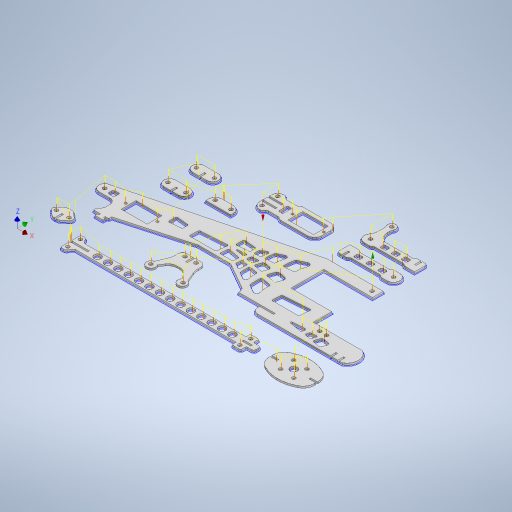
# Autodesk Inventor part: carbon_15
Saved by Autodesk Inventor 2024 (Build 280153000, 153)
## iProperties
Created: 2024-04-23
Part Number: carbon_15
Material: Generic
Document SubType Name: Modeling
Designer: nikop
Density: 1 g/cm^3
Appearance: Default
Author: nikop
Autodesk Inventor part; units mm, degrees
(part 1 of 2)
ref_plane "YZ Plane" through (0, 0, 0) normal (1, 0, 0) x (0, 1, 0)
ref_plane "XZ Plane" through (0, 0, 0) normal (0, 1, 0) x (-1, 0, 0)
ref_plane "XY Plane" through (0, 0, 0) normal (0, 0, 1) x (1, 0, 0)
sketch "Sketch2" plane through (0, 0, 0) normal (0, 1, 0) x (-1, 0, 0)
  line L0 (63.9659, -21.9846) -> (63.9659, -21.2726)
  line L1 (42.3159, -21.2726) -> (42.3159, -21.9846)
  arc A0 (42.3159, -21.9846) -> (48.3159, -27.9846) centre (48.3159, -21.9846) ccw
  line L2 (48.3159, -27.9846) -> (57.9659, -27.9846)
  arc A1 (57.9659, -27.9846) -> (63.9659, -21.9846) centre (57.9659, -21.9846) ccw
  line L3 (114.4342, 45.8312) -> (115.9235, 45.8312)
  line L4 (115.9235, 45.8312) -> (117.4264, 45.8275)
  line L5 (32.988, -58.0785) -> (33.7, -58.0785)
  arc A2 (33.7, -58.0785) -> (39.7, -52.0785) centre (33.7, -52.0785) ccw
  arc A3 (39.7, -42.4285) -> (33.7, -36.4285) centre (33.7, -42.4285) ccw
  line L6 (33.7, -36.4285) -> (32.988, -36.4285)
  line L7 (-8.55, -41.8285) -> (-8.55, -47.2535)
  line L8 (-8.55, -47.2535) -> (-8.55, -52.6785)
  line L9 (32.988, -58.0785) -> (31.0417, -56.1321)
  line L10 (-6.9772, -57.0785) -> (16.4833, -57.0785)
  line L11 (18.6047, -56.1998) -> (18.6723, -56.1321)
  line L12 (27.488, -55.2535) -> (28.9204, -55.2535)
  line L13 (27.488, -55.2535) -> (20.7936, -55.2535)
  line L14 (-12.85, -47.2535) -> (-12.85, -51.3363)
  line L15 (-11.5744, -54.265) -> (-9.7016, -56.0072)
  arc A4 (-12.85, -51.3363) -> (-11.5744, -54.265) centre (-8.85, -51.3363) ccw
  arc A5 (-9.7016, -56.0072) -> (-6.9772, -57.0785) centre (-6.9772, -53.0785) ccw
  arc A6 (31.0417, -56.1321) -> (28.9204, -55.2535) centre (28.9204, -58.2535) ccw
  arc A7 (20.7936, -55.2535) -> (18.6723, -56.1321) centre (20.7936, -58.2535) ccw
  arc A8 (16.4833, -57.0785) -> (18.6047, -56.1998) centre (16.4833, -54.0785) ccw
  line L16 (32.988, -36.4285) -> (31.0417, -38.3748)
  line L17 (-6.9772, -37.4285) -> (16.4833, -37.4285)
  line L18 (18.6047, -38.3071) -> (18.6723, -38.3748)
  line L19 (27.488, -39.2535) -> (28.9204, -39.2535)
  line L20 (27.488, -39.2535) -> (20.7936, -39.2535)
  line L21 (-12.85, -47.2535) -> (-12.85, -43.1706)
  line L22 (-11.5744, -40.2419) -> (-9.7016, -38.4997)
  arc A9 (-11.5744, -40.2419) -> (-12.85, -43.1706) centre (-8.85, -43.1706) ccw
  arc A10 (-6.9772, -37.4285) -> (-9.7016, -38.4997) centre (-6.9772, -41.4285) ccw
  arc A11 (28.9204, -39.2535) -> (31.0417, -38.3748) centre (28.9204, -36.2535) ccw
  arc A12 (18.6723, -38.3748) -> (20.7936, -39.2535) centre (20.7936, -36.2535) ccw
  arc A13 (18.6047, -38.3071) -> (16.4833, -37.4285) centre (16.4833, -40.4285) ccw
  line L23 (23.488, -51.2535) -> (21.55, -51.2535)
  line L24 (20.55, -50.2535) -> (20.55, -44.2535)
  line L25 (24.488, -50.2535) -> (24.488, -44.2535)
  line L26 (23.488, -43.2535) -> (21.55, -43.2535)
  arc A14 (23.488, -51.2535) -> (24.488, -50.2535) centre (23.488, -50.2535) ccw
  arc A15 (20.55, -50.2535) -> (21.55, -51.2535) centre (21.55, -50.2535) ccw
  arc A16 (21.55, -43.2535) -> (20.55, -44.2535) centre (21.55, -44.2535) ccw
  arc A17 (24.488, -44.2535) -> (23.488, -43.2535) centre (23.488, -44.2535) ccw
  arc A18 (-39.6917, -79.1119) -> (-39.0716, -76.4297) centre (-45.0715, -76.4553) ccw
  arc A19 (-39.6917, -79.1119) -> (-33.443, -79.1097) centre (-36.5668, -80.6883) ccw
  arc A20 (-34.0716, -76.4362) -> (-33.443, -79.1097) centre (-28.0716, -76.4362) ccw
  arc A21 (-32.1328, -65.5122) -> (-34.0716, -71.4122) centre (-24.1248, -71.4122) ccw
  arc A22 (-32.1328, -65.5122) -> (-36.5683, -56.76) centre (-36.5683, -62.26) ccw
  line L27 (-36.5683, -56.76) -> (-41.2399, -56.76)
  arc A23 (-41.2399, -56.76) -> (-42.6541, -57.3458) centre (-41.2399, -58.76) ccw
  line L28 (-42.6541, -57.3458) -> (-42.9825, -57.6743)
  arc A24 (-44.3967, -58.26) -> (-42.9825, -57.6743) centre (-44.3967, -56.26) ccw
  line L29 (-69.3967, -58.26) -> (-71.0483, -57.3065)
  arc A25 (-71.0483, -57.3065) -> (-72.5112, -56.805) centre (-72.378, -58.8005) ccw
  line L30 (-72.5112, -56.805) -> (-78.1828, -56.805)
  arc A26 (-72.5112, -67.805) -> (-71.097, -67.2192) centre (-72.5112, -65.805) ccw
  line L31 (-71.097, -67.2192) -> (-70.7686, -66.8907)
  arc A27 (-69.3967, -66.26) -> (-70.7686, -66.8907) centre (-69.309, -68.2581) ccw
  arc A28 (-42.9825, -66.8458) -> (-44.3967, -66.26) centre (-44.3967, -68.26) ccw
  line L32 (-42.9825, -66.8458) -> (-41.9972, -67.8311)
  arc A29 (-39.0716, -74.8989) -> (-41.9972, -67.8311) centre (-49.0716, -74.8989) ccw
  arc A30 (-68.7467, -39.07) -> (-67.3325, -39.6557) centre (-67.3325, -37.6557) ccw
  line L33 (-68.7467, -39.07) -> (-69.0752, -38.7415)
  arc A31 (-69.0752, -38.7415) -> (-70.4894, -38.1557) centre (-70.4894, -40.1557) ccw
  line L34 (-70.4894, -38.1557) -> (-75.1609, -38.1557)
  arc A32 (-75.1609, -38.1557) -> (-80.6609, -43.6557) centre (-75.1609, -43.6557) ccw
  arc A33 (-80.6609, -43.6557) -> (-75.1609, -49.1557) centre (-75.1609, -43.6557) ccw
  line L35 (-75.1609, -49.1557) -> (-70.4894, -49.1557)
  arc A34 (-70.4894, -49.1557) -> (-69.0752, -48.57) centre (-70.4894, -47.1557) ccw
  line L36 (-69.0752, -48.57) -> (-68.7467, -48.2415)
  arc A35 (-67.3325, -47.6557) -> (-68.7467, -48.2415) centre (-67.3325, -49.6557) ccw
  arc A36 (-41.2081, -48.1834) -> (-42.3325, -47.6557) centre (-42.578, -49.6406) ccw
  line L37 (-41.2081, -48.1834) -> (-40.8797, -48.5118)
  arc A37 (-40.8797, -48.5118) -> (-39.4655, -49.0976) centre (-39.4655, -47.0976) ccw
  line L38 (-39.4655, -49.0976) -> (-33.7939, -49.0976)
  arc A38 (-39.4655, -38.0976) -> (-40.8797, -38.6834) centre (-39.4655, -40.0976) ccw
  line L39 (-40.8797, -38.6834) -> (-41.2081, -39.0118)
  arc A39 (-42.3325, -39.6557) -> (-41.2081, -39.0118) centre (-42.7106, -37.6918) ccw
  line L40 (-56.1358, -62.2237) -> (-56.1358, -63.2237)
  line L41 (-56.1358, -62.2237) -> (-56.1358, -61.2237)
  line L42 (-69.7689, -62.305) -> (-69.7689, -63.305)
  line L43 (-69.7689, -62.305) -> (-69.7689, -61.305)
  line L44 (-65.7689, -60.305) -> (-68.7689, -60.305)
  line L45 (-80.1828, -62.305) -> (-80.1828, -65.805)
  line L46 (-80.1828, -62.305) -> (-80.1828, -58.805)
  arc A40 (-80.1828, -65.805) -> (-78.1828, -67.805) centre (-78.1828, -65.805) ccw
  arc A41 (-69.7689, -63.305) -> (-68.7689, -64.305) centre (-68.7689, -63.305) ccw
  arc A42 (-68.7689, -60.305) -> (-69.7689, -61.305) centre (-68.7689, -61.305) ccw
  arc A43 (-57.1358, -64.2237) -> (-56.1358, -63.2237) centre (-57.1358, -63.2237) ccw
  arc A44 (-56.1358, -61.2237) -> (-57.1358, -60.2237) centre (-57.1358, -61.2237) ccw
  line L47 (-68.7689, -64.305) -> (-65.7689, -64.305)
  line L48 (-64.7689, -61.305) -> (-64.7689, -63.305)
  line L49 (-61.1358, -61.2237) -> (-61.1358, -63.2237)
  line L50 (-60.1358, -64.2237) -> (-57.1358, -64.2237)
  line L51 (-60.1358, -60.2237) -> (-57.1358, -60.2237)
  arc A45 (-65.7689, -64.305) -> (-64.7689, -63.305) centre (-65.7689, -63.305) ccw
  arc A46 (-64.7689, -61.305) -> (-65.7689, -60.305) centre (-65.7689, -61.305) ccw
  arc A47 (-61.1358, -63.2237) -> (-60.1358, -64.2237) centre (-60.1358, -63.2237) ccw
  arc A48 (-60.1358, -60.2237) -> (-61.1358, -61.2237) centre (-60.1358, -61.2237) ccw
  line L52 (-31.7939, -43.5976) -> (-31.7939, -40.0976)
  line L53 (-31.7939, -43.5976) -> (-31.7939, -47.0976)
  arc A49 (-31.7939, -40.0976) -> (-33.7939, -38.0976) centre (-33.7939, -40.0976) ccw
  line L54 (-67.9654, -43.7185) -> (-67.9654, -42.7185)
  line L55 (-67.9654, -43.7185) -> (-67.9654, -44.7185)
  line L56 (-42.268, -43.5976) -> (-42.268, -42.5976)
  line L57 (-42.268, -43.5976) -> (-42.268, -44.5976)
  line L58 (-46.268, -45.5976) -> (-43.268, -45.5976)
  arc A50 (-42.268, -42.5976) -> (-43.268, -41.5976) centre (-43.268, -42.5976) ccw
  arc A51 (-43.268, -45.5976) -> (-42.268, -44.5976) centre (-43.268, -44.5976) ccw
  arc A52 (-66.9654, -41.7185) -> (-67.9654, -42.7185) centre (-66.9654, -42.7185) ccw
  arc A53 (-67.9654, -44.7185) -> (-66.9654, -45.7185) centre (-66.9654, -44.7185) ccw
  line L59 (-43.268, -41.5976) -> (-46.268, -41.5976)
  line L60 (-47.268, -44.5976) -> (-47.268, -42.5976)
  line L61 (-62.9654, -44.7185) -> (-62.9654, -42.7185)
  line L62 (-63.9654, -41.7185) -> (-66.9654, -41.7185)
  line L63 (-63.9654, -45.7185) -> (-66.9654, -45.7185)
  arc A54 (-46.268, -41.5976) -> (-47.268, -42.5976) centre (-46.268, -42.5976) ccw
  arc A55 (-47.268, -44.5976) -> (-46.268, -45.5976) centre (-46.268, -44.5976) ccw
  arc A56 (-62.9654, -42.7185) -> (-63.9654, -41.7185) centre (-63.9654, -42.7185) ccw
  arc A57 (-63.9654, -45.7185) -> (-62.9654, -44.7185) centre (-63.9654, -44.7185) ccw
  line L64 (-63.4368, 73.5321) -> (-63.4368, 73.3321)
  arc A58 (-64.4368, 72.3321) -> (-63.4368, 73.3321) centre (-64.4368, 73.3321) ccw
  line L65 (-64.4368, 72.3321) -> (-67.9559, 72.3321)
  arc A59 (-67.9559, 72.3321) -> (-69.9559, 70.3321) centre (-67.9559, 70.3321) ccw
  line L66 (-69.9559, 70.3321) -> (-69.9559, 68.3321)
  arc A60 (-69.9559, 68.3321) -> (-67.9559, 66.3321) centre (-67.9559, 68.3321) ccw
  line L67 (-67.9559, 66.3321) -> (-64.4368, 66.3321)
  arc A61 (-63.4193, 65.3322) -> (-64.4368, 66.3321) centre (-64.4193, 65.3322) ccw
  line L68 (-63.4193, 65.3322) -> (-63.4193, 65.1321)
  line L69 (121.1391, 17.6529) -> (121.1391, 17.654)
  line L70 (4.289, 17.6186) -> (-16.8908, 29.6804)
  line L71 (105.5881, 35.3778) -> (105.5881, 34.2063)
  arc A62 (116.9799, 9.8778) -> (121.9799, 14.8778) centre (116.9799, 14.8778) ccw
  line L72 (105.0881, 35.8778) -> (99.4807, 35.8778)
  line L73 (95.4807, 37.4038) -> (94.2807, 37.4038)
  line L74 (100.6807, 37.4038) -> (99.4807, 37.4038)
  line L75 (93.9807, 37.7038) -> (93.9807, 39.1038)
  line L76 (100.9807, 37.7038) -> (100.9807, 39.1038)
  line L77 (95.4791, 37.4038) -> (94.2791, 37.4028)
  arc A63 (93.9807, 37.7038) -> (94.2807, 37.4038) centre (94.2807, 37.7038) ccw
  arc A64 (94.2807, 39.4038) -> (93.9807, 39.1038) centre (94.2807, 39.1038) ccw
  arc A65 (100.9807, 39.1038) -> (100.6807, 39.4038) centre (100.6807, 39.1038) ccw
  arc A66 (100.6807, 37.4038) -> (100.9807, 37.7038) centre (100.6807, 37.7038) ccw
  arc A67 (121.9799, 14.8778) -> (116.9799, 19.8778) centre (116.9799, 14.8778) ccw
  line L78 (116.9799, 19.8778) -> (107.4799, 19.8778)
  line L79 (105.5881, 35.3778) -> (105.5881, 34.8778)
  line L80 (105.0023, 32.792) -> (103.9444, 31.7341)
  line L81 (102.4799, 24.8778) -> (102.4799, 28.1985)
  arc A68 (103.9444, 31.7341) -> (102.4799, 28.1985) centre (107.4799, 28.1985) ccw
  arc A69 (102.4799, 24.8778) -> (107.4799, 19.8778) centre (107.4799, 24.8778) ccw
  arc A70 (105.0023, 32.792) -> (105.5881, 34.2063) centre (103.5881, 34.2063) ccw
  line L82 (92.4791, 35.3778) -> (92.4791, 33.2966)
  line L83 (92.9791, 35.8778) -> (95.4791, 35.8778)
  arc A71 (92.9791, 35.8778) -> (92.4791, 35.3778) centre (92.9791, 35.3778) ccw
  arc A72 (105.5881, 35.3778) -> (105.0881, 35.8778) centre (105.0881, 35.3778) ccw
  arc A73 (-19.2582, 33.8243) -> (-16.8908, 29.6804) centre (-14.2593, 33.9319) ccw
  arc A74 (112.0363, 15.6265) -> (112.0363, 14.1292) centre (116.9799, 14.8778) ccw
  line L84 (-9.9813, 1.6568) -> (-13.6957, 2.4536)
  arc A75 (-15.0721, 5.2892) -> (-13.7944, 8.5218) centre (-34.7824, 14.9487) ccw
  arc A76 (4.289, 17.6186) -> (6.789, 16.9487) centre (6.789, 21.9487) ccw
  arc A77 (-15.0721, 5.2892) -> (-13.6957, 2.4536) centre (-13.2762, 4.4091) ccw
  arc A78 (-10.6169, 22.7604) -> (-13.5514, 20.5207) centre (-11.6169, 21.0284) ccw
  line L85 (110.663, 17.3471) -> (107.4546, 17.5827)
  arc A79 (110.663, 12.4086) -> (112.0363, 14.1292) centre (110.5532, 13.9046) ccw
  arc A80 (112.0363, 15.6265) -> (110.663, 17.3471) centre (110.5532, 15.8511) ccw
  line L86 (110.663, 12.4086) -> (107.4546, 12.173)
  arc A81 (107.4546, 17.5827) -> (106.3814, 16.5854) centre (107.3814, 16.5854) ccw
  arc A82 (106.3814, 13.1703) -> (107.4546, 12.173) centre (107.3814, 13.1703) ccw
  line L87 (110.663, 12.4086) -> (107.4546, 12.173)
  line L88 (-8.4093, 1.7319) -> (-9.6983, 1.6372)
  line L89 (-8.4093, 1.7319) -> (-9.6983, 1.6372)
  line L90 (0.9741, 2.4209) -> (-3.375, 2.1015)
  line L91 (0.9741, 2.4209) -> (-3.375, 2.1015)
  line L92 (0.9741, 2.4209) -> (-3.375, 2.1015)
  line L93 (0.9741, 2.4209) -> (-3.375, 2.1015)
  line L94 (0.9741, 2.4209) -> (-3.375, 2.1015)
  line L95 (0.9741, 2.4209) -> (-3.375, 2.1015)
  line L96 (0.9741, 2.4209) -> (-3.375, 2.1015)
  line L97 (0.9741, 2.4209) -> (-3.375, 2.1015)
  line L98 (0.9741, 2.4209) -> (-3.375, 2.1015)
  line L99 (0.9741, 2.4209) -> (-3.375, 2.1015)
  line L100 (-8.4093, 1.7319) -> (-9.6983, 1.6372)
  line L101 (-8.4093, 1.7319) -> (-9.6983, 1.6372)
  line L102 (-8.4093, 1.7319) -> (-9.6983, 1.6372)
  line L103 (-8.4093, 1.7319) -> (-9.6983, 1.6372)
  line L104 (-8.4093, 1.7319) -> (-9.6983, 1.6372)
  line L105 (-8.4093, 1.7319) -> (-9.6983, 1.6372)
  line L106 (-8.4093, 1.7319) -> (-9.6983, 1.6372)
  line L107 (-8.4093, 1.7319) -> (-9.6983, 1.6372)
  line L108 (16.896, 3.5901) -> (16.8305, 3.5853)
  line L109 (16.896, 3.5901) -> (16.8305, 3.5853)
  line L110 (16.896, 3.5901) -> (16.8305, 3.5853)
  line L111 (16.896, 3.5901) -> (16.8305, 3.5853)
  line L112 (16.896, 3.5901) -> (16.8305, 3.5853)
  line L113 (16.896, 3.5901) -> (16.8305, 3.5853)
  line L114 (16.896, 3.5901) -> (16.8305, 3.5853)
  line L115 (16.896, 3.5901) -> (16.8305, 3.5853)
  line L116 (16.896, 3.5901) -> (16.8305, 3.5853)
  line L117 (13.1011, 3.3114) -> (6.3051, 2.8124)
  line L118 (43.3602, 5.5334) -> (25.7785, 4.2424)
  line L119 (43.3602, 5.5334) -> (25.7785, 4.2424)
  line L120 (43.3602, 5.5334) -> (25.7785, 4.2424)
  line L121 (43.3602, 5.5334) -> (25.7785, 4.2424)
  line L122 (43.3602, 5.5334) -> (25.7785, 4.2424)
  line L123 (43.3602, 5.5334) -> (25.7785, 4.2424)
  line L124 (43.3602, 5.5334) -> (25.7785, 4.2424)
  line L125 (43.3602, 5.5334) -> (25.7785, 4.2424)
  line L126 (43.3602, 5.5334) -> (25.7785, 4.2424)
  line L127 (43.3602, 5.5334) -> (21.4119, 3.9217)
  line L128 (6.6161, 5.5458) -> (13.1579, 4.3013)
  line L129 (-2.2448, 7.2316) -> (1.6945, 6.4821)
  line L130 (-12.6513, 9.2114) -> (-6.6798, 8.0753)
  line L131 (7.1768, 8.493) -> (16.5175, 6.7159)
  line L132 (-1.6841, 10.1787) -> (2.2552, 9.4293)
  line L133 (-12.0906, 12.1585) -> (-6.1191, 11.0225)
  arc A83 (-12.9006, 13.2197) -> (-13.5514, 20.5207) centre (-34.7824, 14.9487) ccw
  arc A84 (-12.9006, 13.2197) -> (-12.0906, 12.1585) centre (-11.9037, 13.1409) ccw
  arc A85 (-12.6513, 9.2114) -> (-13.7944, 8.5218) centre (-12.8382, 8.229) ccw
  arc A86 (-5.9041, 6.8221) -> (-6.6798, 8.0753) centre (-6.8667, 7.093) ccw
  arc A87 (-9.9813, 1.6568) -> (-9.6983, 1.6372) centre (-9.7716, 2.6345) ccw
  arc A88 (-8.4093, 1.7319) -> (-7.5757, 2.3078) centre (-8.4826, 2.7292) ccw
  arc A89 (-4.3836, 3.4526) -> (-3.375, 2.1015) centre (-3.4482, 3.0989) ccw
  arc A90 (-2.2448, 7.2316) -> (-3.3974, 6.5089) centre (-2.4317, 6.2492) ccw
  arc A91 (2.4754, 5.2478) -> (1.6945, 6.4821) centre (1.5076, 5.4998) ccw
  arc A92 (0.9741, 2.4209) -> (1.8524, 3.1107) centre (0.9009, 3.4182) ccw
  arc A93 (5.2668, 4.0718) -> (6.3051, 2.8124) centre (6.2319, 3.8097) ccw
  arc A94 (6.6161, 5.5458) -> (5.4595, 4.8078) centre (6.4292, 4.5635) ccw
  arc A95 (-2.4908, 11.2742) -> (-1.6841, 10.1787) centre (-1.4972, 11.1611) ccw
  arc A96 (2.2552, 9.4293) -> (3.4347, 10.2907) centre (2.4421, 10.4117) ccw
  arc A97 (3.7029, 13.8877) -> (3.2033, 14.7813) centre (2.7033, 13.9153) ccw
  arc A98 (-0.807, 17.0967) -> (-2.3062, 16.1924) centre (-1.307, 16.2306) ccw
  arc A99 (-5.0732, 19.1157) -> (-5.5636, 19.8429) centre (-6.0636, 18.9768) ccw
  arc A100 (7.6705, 13.9487) -> (6.6716, 12.9958) centre (7.6705, 12.9487) ccw
  arc A101 (18.166, 12.9067) -> (17.1668, 13.9487) centre (17.1668, 12.9487) ccw
  arc A102 (16.5175, 6.7159) -> (17.6954, 7.565) centre (16.7044, 7.6983) ccw
  arc A103 (-6.1191, 11.0225) -> (-4.9374, 11.9034) centre (-5.9322, 12.0049) ccw
  arc A104 (13.1011, 3.3114) -> (13.1579, 4.3013) centre (13.0644, 3.8101) ccw
  line L134 (13.1011, 3.3114) -> (6.3051, 2.8124)
  line L135 (13.1011, 3.3114) -> (6.3051, 2.8124)
  line L136 (13.1011, 3.3114) -> (6.3051, 2.8124)
  line L137 (13.1011, 3.3114) -> (6.3051, 2.8124)
  line L138 (13.1011, 3.3114) -> (6.3051, 2.8124)
  line L139 (13.1011, 3.3114) -> (6.3051, 2.8124)
  line L140 (13.1011, 3.3114) -> (6.3051, 2.8124)
  line L141 (13.1011, 3.3114) -> (6.3051, 2.8124)
  line L142 (13.1011, 3.3114) -> (6.3051, 2.8124)
  line L143 (23.709, 13.9487) -> (22.1709, 13.9487)
  line L144 (17.1668, 13.9487) -> (7.6705, 13.9487)
  arc A105 (6.372, 9.6041) -> (7.1768, 8.493) centre (7.3637, 9.4754) ccw
  line L145 (43.6933, 13.9487) -> (23.709, 13.9487)
  arc A106 (22.1709, 13.9487) -> (21.1717, 12.9873) centre (22.1709, 12.9487) ccw
  arc A107 (20.3528, 5.0861) -> (21.4119, 3.9217) centre (21.3387, 4.919) ccw
  arc A108 (43.3602, 5.5334) -> (44.2818, 6.4287) centre (43.287, 6.5307) ccw
  arc A109 (44.693, 12.9245) -> (43.6933, 13.9487) centre (43.6933, 12.9487) ccw
  line L146 (3.2033, 14.7813) -> (-0.807, 17.0967)
  line L147 (-5.5636, 19.8429) -> (-10.6169, 22.7604)
  line L148 (106.3814, 16.5854) -> (106.3814, 13.1703)
  arc A110 (-7.5757, 2.3078) -> (-5.9041, 6.8221) centre (-34.7824, 14.9487) ccw
  arc A111 (-4.9374, 11.9034) -> (-5.0732, 19.1157) centre (-34.7824, 14.9487) ccw
  arc A112 (-4.3836, 3.4526) -> (-3.3974, 6.5089) centre (-34.7824, 14.9487) ccw
  arc A113 (-2.4908, 11.2742) -> (-2.3062, 16.1924) centre (-34.7824, 14.9487) ccw
  arc A114 (17.6954, 7.565) -> (18.166, 12.9067) centre (-40.2824, 15.3634) ccw
  arc A115 (20.3528, 5.0861) -> (21.1717, 12.9873) centre (-40.2824, 15.3634) ccw
  arc A116 (21.185, 17.3634) -> (21.1834, 17.4134) centre (-40.2824, 15.3634) ccw
  arc A117 (44.2818, 6.4287) -> (44.693, 12.9245) centre (-38.7824, 14.9487) ccw
  arc A118 (47.6944, 16.9717) -> (47.6935, 17.007) centre (-38.7825, 14.9717) ccw
  arc A119 (1.8524, 3.1107) -> (2.4754, 5.2478) centre (-34.7824, 14.9487) ccw
  arc A120 (3.4347, 10.2907) -> (3.7029, 13.8877) centre (-34.7824, 14.9487) ccw
  arc A121 (3.7148, 14.486) -> (3.7149, 14.4939) centre (-34.7824, 14.9487) ccw
  arc A122 (5.2668, 4.0718) -> (5.4595, 4.8078) centre (-34.7824, 14.9487) ccw
  arc A123 (6.372, 9.6041) -> (6.6716, 12.9958) centre (-34.7824, 14.9487) ccw
  line L149 (18.1699, 45.3626) -> (15.4569, 49.3848)
  line L150 (33.8183, 45.3626) -> (36.5313, 49.3848)
  line L151 (25.9941, 41.8361) -> (24.8022, 41.8361)
  line L152 (25.9941, 41.8361) -> (27.186, 41.8361)
  arc A124 (18.1699, 45.3626) -> (24.8022, 41.8361) centre (24.8022, 49.8361) ccw
  arc A125 (27.186, 41.8361) -> (33.8183, 45.3626) centre (27.186, 49.8361) ccw
  circle A126 centre (11.9941, 51.8361) radius 1.55
  circle A127 centre (39.9941, 51.8361) radius 1.55
  line L153 (94.2807, 39.4038) -> (100.6807, 39.4038)
  line L154 (-19.2582, 33.9482) -> (-19.2582, 33.8243)
  line L155 (89.0441, 65.8321) -> (89.3041, 65.8321) construction
  line L156 (92.0263, 66.8987) -> (92.0263, 61.3987)
  arc A128 (89.5263, 60.3987) -> (92.0263, 61.3987) centre (89.7806, 63.3879) ccw
  arc A129 (87.0263, 61.3987) -> (89.5263, 60.3987) centre (89.272, 63.3879) ccw
  line L157 (92.0419, 71.8659) -> (92.0419, 77.3659)
  arc A130 (92.0419, 77.3659) -> (89.5419, 78.3659) centre (89.7962, 75.3767) ccw
  arc A131 (89.5419, 78.3659) -> (87.0263, 77.3481) centre (89.2876, 75.3767) ccw
  arc A132 (119.3083, 58.1434) -> (117.4289, 58.8275) centre (117.4012, 55.8276) ccw
  arc A133 (117.4264, 45.8275) -> (119.3058, 46.5115) centre (117.3988, 48.8273) ccw
  arc A134 (114.4127, 58.8312) -> (112.5333, 58.1472) centre (114.4404, 55.8313) ccw
  arc A135 (112.5549, 46.5152) -> (114.4342, 45.8312) centre (114.4619, 48.8311) ccw
  line L158 (-55.8664, 73.4812) -> (84.1336, 73.4812)
  line L159 (-55.8758, 65.1984) -> (84.1242, 65.1984)
  line L160 (83.9404, -12.0118) -> (84.7029, -12.0118)
  line L161 (87.7029, -12.0118) -> (88.4653, -12.0118)
  circle A136 centre (89.0441, 74.8321) radius 1.55
  circle A137 centre (89.0441, 63.8321) radius 1.55
  arc A138 (87.0263, 61.3987) -> (84.1242, 65.1984) centre (79.508, 58.6647) ccw
  arc A139 (84.1336, 73.4812) -> (87.0263, 77.3481) centre (79.4727, 79.9832) ccw
  circle A140 centre (-59.4485, 74.0821) radius 1.55
  circle A141 centre (-59.4562, 64.5821) radius 1.55
  line L162 (-63.4193, 65.1321) -> (-63.4193, 62.1321)
  arc A142 (-63.4193, 62.1321) -> (-61.5716, 61.3667) centre (-61.8326, 63.3496) ccw
  line L163 (-55.8758, 65.1984) -> (-55.8758, 62.1321)
  arc A143 (-57.7235, 61.3667) -> (-55.8758, 62.1321) centre (-57.4625, 63.3496) ccw
  line L164 (-61.5716, 61.3667) -> (-57.7235, 61.3667)
  line L165 (-63.4368, 73.5321) -> (-63.4368, 76.5321)
  line L166 (-55.8664, 73.4812) -> (-55.8664, 76.5321)
  arc A144 (-55.8664, 76.5321) -> (-57.7142, 77.2974) centre (-57.4531, 75.3146) ccw
  arc A145 (-61.589, 77.2974) -> (-63.4368, 76.5321) centre (-61.8501, 75.3146) ccw
  line L167 (-61.589, 77.2974) -> (-57.7142, 77.2974)
  circle A146 centre (21.2441, 31.3361) radius 1.55
  circle A147 centre (30.7441, 31.3361) radius 1.55
  line L168 (24.4941, 28.3361) -> (19.4941, 28.3361)
  arc A148 (15.9585, 31.8717) -> (19.4941, 28.3361) centre (19.9343, 32.3118) ccw
  line L169 (15.9585, 31.8717) -> (15.9585, 34.8717)
  arc A149 (15.9585, 34.8717) -> (14.9831, 39.7756) centre (5.9744, 35.4347) ccw
  line L170 (14.9831, 39.7756) -> (11.5389, 48.0905)
  arc A150 (15.4569, 49.3848) -> (11.5389, 48.0905) centre (12.423, 51.9916) ccw
  circle A151 centre (110.4234, 52.3502) radius 1.55
  circle A152 centre (121.4236, 52.3589) radius 1.55
  line L171 (112.5333, 58.1472) -> (107.937, 54.2904)
  line L172 (112.5549, 46.5152) -> (107.9586, 50.372)
  arc A153 (107.937, 54.2904) -> (107.9586, 50.372) centre (109.5006, 52.3397) ccw
  line L173 (119.3058, 46.5115) -> (123.9021, 50.3682)
  line L174 (119.3083, 58.1434) -> (123.9045, 54.2867)
  arc A154 (123.9021, 50.3682) -> (123.9045, 54.2867) centre (122.3504, 52.3284) ccw
  line L175 (39.7, -52.0785) -> (39.7, -51.7535)
  line L176 (-8.55, -52.6785) -> (-8.55, -53.6785)
  line L177 (-8.55, -41.8285) -> (-8.55, -40.8285)
  line L178 (-8.55, -53.6785) -> (13.65, -53.6785)
  line L179 (-8.55, -40.8285) -> (13.65, -40.8285)
  line L180 (13.65, -53.6785) -> (13.65, -40.8285)
  line L181 (39.7, -42.4285) -> (39.7, -42.7535)
  line L182 (39.7, -48.7535) -> (39.7, -45.7535)
  circle A155 centre (35.788, -40.3535) radius 1.55
  circle A156 centre (35.788, -54.1535) radius 1.55
  circle A157 centre (46.2409, -24.0726) radius 1.55
  circle A158 centre (60.0409, -24.0726) radius 1.55
  line L183 (-72.5112, -67.805) -> (-73.6828, -67.805)
  line L184 (-76.6797, -67.805) -> (-78.1828, -67.805)
  circle A159 centre (-36.5683, -62.26) radius 1.55
  circle A160 centre (-36.5748, -80.6723) radius 1.55
  circle A161 centre (-75.1609, -43.6557) radius 1.55
  line L185 (-33.7939, -38.0976) -> (-35.2939, -38.0976)
  line L186 (-38.2939, -38.0976) -> (-39.4655, -38.0976)
  line L187 (94.0577, 10.5517) -> (71.558, 10.6609)
  line L188 (94.0577, 10.5517) -> (94.0577, 23.4561)
  line L189 (94.0577, 23.4561) -> (71.5577, 23.4556)
  line L190 (71.5577, 23.4556) -> (71.558, 10.6609)
  circle A162 centre (116.9704, 14.938) radius 1.55
  line L191 (-34.0716, -76.4362) -> (-34.0716, -71.4122)
  line L192 (-39.0716, -76.4297) -> (-39.0716, -74.8989)
  circle A163 centre (-106.6787, 63.0954) radius 1.525
  circle A164 centre (-95.365, 74.4091) radius 1.525
  circle A165 centre (-107.7394, 75.4697) radius 1.525
  circle A166 centre (-94.3044, 62.0347) radius 1.525
  line L193 (-44.3967, -66.26) -> (-69.3967, -66.26)
  line L194 (-44.3967, -58.26) -> (-69.3967, -58.26)
  line L195 (-51.7166, -61.152) -> (-51.7166, -63.152)
  line L196 (-50.7166, -60.152) -> (-47.7166, -60.152)
  line L197 (-50.7166, -64.152) -> (-47.7166, -64.152)
  arc A167 (-51.7166, -63.152) -> (-50.7166, -64.152) centre (-50.7166, -63.152) ccw
  arc A168 (-50.7166, -60.152) -> (-51.7166, -61.152) centre (-50.7166, -61.152) ccw
  arc A169 (-47.7166, -64.152) -> (-46.7166, -63.152) centre (-47.7166, -63.152) ccw
  line L198 (-46.7166, -62.152) -> (-46.7166, -63.152)
  line L199 (-46.7166, -62.152) -> (-46.7166, -61.152)
  arc A170 (-46.7166, -61.152) -> (-47.7166, -60.152) centre (-47.7166, -61.152) ccw
  line L200 (-67.3325, -47.6557) -> (-42.3325, -47.6557)
  line L201 (-67.3325, -39.6557) -> (-42.3325, -39.6557)
  line L202 (-52.5769, -43.6799) -> (-52.5769, -42.6799)
  line L203 (-53.5769, -41.6799) -> (-56.5769, -41.6799)
  line L204 (-52.5769, -43.6799) -> (-52.5769, -44.6799)
  arc A171 (-53.5769, -45.6799) -> (-52.5769, -44.6799) centre (-53.5769, -44.6799) ccw
  arc A172 (-52.5769, -42.6799) -> (-53.5769, -41.6799) centre (-53.5769, -42.6799) ccw
  line L205 (-57.5769, -44.6799) -> (-57.5769, -42.6799)
  arc A173 (-57.5769, -44.6799) -> (-56.5769, -45.6799) centre (-56.5769, -44.6799) ccw
  arc A174 (-56.5769, -41.6799) -> (-57.5769, -42.6799) centre (-56.5769, -42.6799) ccw
  line L206 (-56.5769, -45.6799) -> (-53.5769, -45.6799)
  line L207 (-75.2523, 42.9487) -> (-99.2523, 42.9487)
  line L208 (-74.2523, 25.0966) -> (-115.3023, 25.0966)
  line L209 (83.9404, -12.0118) -> (79.9404, -12.0118)
  line L210 (88.4653, -12.0118) -> (92.4653, -12.0118)
  line L211 (88.4653, -12.0118) -> (92.4653, -12.0118) construction
  circle A175 centre (78.4154, -17.0118) radius 1.525
  arc A176 (79.9404, -12.0118) -> (79.9404, -22.0118) centre (79.9404, -17.0118) ccw
  line L212 (79.9404, -22.0118) -> (92.4653, -22.0118)
  arc A177 (92.4653, -22.0118) -> (92.4653, -12.0118) centre (92.4653, -17.0118) ccw
  circle A178 centre (93.9903, -17.0118) radius 1.525
  line L213 (42.3159, -21.2726) -> (42.3159, -19.7726)
  line L214 (63.9659, -21.2726) -> (63.9659, -19.7726)
  line L215 (42.3159, -19.7726) -> (63.9659, -19.7726)
  line L216 (6.789, 16.9487) -> (33.789, 16.9487)
  line L217 (-50.9967, 34.8873) -> (-19.2582, 34.8873)
  line L218 (-19.2582, 34.8873) -> (-19.2582, 33.8243)
  arc A179 (-87.2534, 57.9059) -> (-81.2534, 67.2522) centre (-91.2517, 67.0718) ccw
  arc A180 (-120.7904, 67.2522) -> (-114.7904, 57.9059) centre (-110.792, 67.0718) ccw
  arc A181 (-114.7904, 57.9059) -> (-87.2534, 57.9059) centre (-101.0219, 84.5598) ccw
  arc A182 (-81.2534, 70.2522) -> (-87.2534, 79.5985) centre (-91.2517, 70.4327) ccw
  arc A183 (-114.7904, 79.5985) -> (-120.7904, 70.2522) centre (-110.792, 70.4327) ccw
  arc A184 (-87.2534, 79.5985) -> (-114.7904, 79.5985) centre (-101.0219, 52.9447) ccw
  line L219 (-26.9701, 15.6496) -> (-19.8043, 14.2863)
  arc A185 (-18.5493, 23.9983) -> (-19.1376, 24.8708) centre (-19.7376, 23.8316) ccw
  arc A186 (-19.8043, 14.2863) -> (-18.3863, 15.3434) centre (-19.5801, 15.4652) ccw
  arc A187 (-18.3863, 15.3434) -> (-18.5493, 23.9983) centre (-54.2003, 18.9978) ccw
  line L220 (-19.1376, 24.8708) -> (-25.2017, 28.3719)
  arc A188 (-27.9421, 16.923) -> (-26.9701, 15.6496) centre (-26.7459, 16.8285) ccw
  arc A189 (-27.9421, 16.923) -> (-28.7231, 25.6842) centre (-54.2003, 18.9978) ccw
  arc A190 (-25.2017, 28.3719) -> (-28.7231, 25.6842) centre (-26.4017, 26.2934) ccw
  line L221 (-21.5647, 2.7268) -> (-23.1115, 2.6132)
  line L222 (-21.5647, 2.7268) -> (-23.1115, 2.6132)
  line L223 (-21.5647, 2.7268) -> (-23.1115, 2.6132)
  line L224 (-21.5647, 2.7268) -> (-23.1115, 2.6132)
  line L225 (-26.6551, 11.7022) -> (-19.4892, 10.339)
  line L226 (-21.5647, 2.7268) -> (-23.1115, 2.6132)
  line L227 (-23.451, 2.6367) -> (-27.9083, 3.5928)
  arc A191 (-29.56, 6.9956) -> (-27.9083, 3.5928) centre (-27.4049, 5.9395) ccw
  arc A192 (-29.56, 6.9956) -> (-28.0267, 10.8747) centre (-53.2124, 18.587) ccw
  line L228 (-21.5647, 2.7268) -> (-23.1115, 2.6132)
  line L229 (-21.5647, 2.7268) -> (-23.1115, 2.6132)
  line L230 (-21.5647, 2.7268) -> (-23.1115, 2.6132)
  line L231 (-21.5647, 2.7268) -> (-23.1115, 2.6132)
  line L232 (-21.5647, 2.7268) -> (-23.1115, 2.6132)
  arc A193 (-20.5643, 3.4179) -> (-18.5584, 8.835) centre (-53.2124, 18.587) ccw
  arc A194 (-21.5647, 2.7268) -> (-20.5643, 3.4179) centre (-21.6525, 3.9236) ccw
  arc A195 (-18.5584, 8.835) -> (-19.4892, 10.339) centre (-19.7135, 9.1601) ccw
  arc A196 (-23.451, 2.6367) -> (-23.1115, 2.6132) centre (-23.1993, 3.81) ccw
  arc A197 (-26.6551, 11.7022) -> (-28.0267, 10.8747) centre (-26.8793, 10.5234) ccw
  circle A198 centre (-101.0219, 68.7522) radius 3
  line L233 (-74.2523, 25.0966) -> (-81.7523, 25.0966)
  line L234 (-74.2523, 25.0966) -> (-81.7523, 25.0966)
  line L235 (-78.1828, -56.805) -> (-80.1828, -56.805)
  line L236 (-80.1828, -56.805) -> (-80.1828, -58.805)
  line L237 (-33.7939, -49.0976) -> (-31.7939, -49.0976)
  line L238 (-33.7939, -49.0976) -> (-35.7939, -49.0976) construction
  line L239 (-31.7939, -49.0976) -> (-31.7939, -47.0976)
  arc A199 (-38.9967, 37.8873) -> (-44.058, 42.9487) centre (-43.9963, 37.9491) ccw
  line L240 (-75.2523, 42.9487) -> (-44.058, 42.9487)
  line L241 (-73.7828, -67.805) -> (-73.6828, -67.805)
  line L242 (-76.5828, -67.805) -> (-76.6797, -67.805)
  line L243 (-38.1939, -38.0976) -> (-38.2939, -38.0976)
  line L244 (-35.3939, -38.0976) -> (-35.2939, -38.0976)
  line L245 (-101.2523, 42.9487) -> (-99.2523, 42.9487)
  circle A200 centre (-89.7523, 29.0966) radius 1.525
  circle A201 centre (-83.7523, 29.0966) radius 1.525
  line L246 (-101.2523, 42.9487) -> (-99.2523, 42.9487) construction
  circle A202 centre (16.1, -47.2535) radius 1.05
  circle A203 centre (-11, -47.2535) radius 1.05
  line L247 (-101.2523, 42.9487) -> (-105.2523, 42.9487)
  line L248 (-101.2523, 42.9487) -> (-97.2523, 42.9487) construction
  line L249 (-108.2523, 37.9487) -> (-108.2523, 42.9487)
  line L250 (-108.2523, 42.9487) -> (-113.2523, 42.9487)
  line L251 (-113.2523, 42.9487) -> (-113.2523, 37.9487)
  line L252 (-115.2523, 42.9487) -> (-117.2523, 42.9487)
  line L253 (-115.3023, 25.0966) -> (-116.7523, 25.0966)
  arc A204 (-117.2523, 42.9487) -> (-116.7523, 25.0966) centre (-112.5027, 34.1487) ccw
  circle A205 centre (96.5577, 17.0039) radius 1.05
  circle A206 centre (69.0579, 17.0583) radius 1.05
  line L254 (-81.2523, -28.5336) -> (-32.4689, -28.5336)
  line L255 (-81.2523, -28.5336) -> (-81.2523, -19.2616)
  line L256 (-81.2523, -19.2616) -> (-38.9967, -19.2616)
  circle A207 centre (-76.2523, -23.8976) radius 1.525
  line L257 (-74.2523, 25.0966) -> (-74.2523, 10.0966)
  line L258 (-74.2523, 10.0966) -> (-74.2523, 9.0966)
  line L259 (-74.2523, 10.0966) -> (-73.2523, 10.0966) construction
  line L260 (-74.2523, 9.0966) -> (-38.9967, 9.0966)
  line L261 (-38.9967, 9.0966) -> (-38.9967, -19.2616)
  circle A208 centre (68.6445, 69.3321) radius 3
  circle A209 centre (59.6445, 69.3321) radius 3
  circle A210 centre (50.6445, 69.3321) radius 3
  circle A211 centre (41.6445, 69.3321) radius 3
  circle A212 centre (32.6445, 69.3321) radius 3
  circle A213 centre (23.6445, 69.3321) radius 3
  circle A214 centre (14.6445, 69.3321) radius 3
  circle A215 centre (5.6445, 69.3321) radius 3
  circle A216 centre (-3.3555, 69.3321) radius 3
  circle A217 centre (-12.3555, 69.3321) radius 3
  circle A218 centre (-21.3555, 69.3321) radius 3
  circle A219 centre (-30.3555, 69.3321) radius 3
  circle A220 centre (-39.3555, 69.3321) radius 3
  circle A221 centre (-48.3555, 69.3321) radius 3
  line L262 (-27.4398, -4.4554) -> (-20.1796, -3.7505)
  arc A222 (-27.4398, -4.4554) -> (-28.5237, -5.635) centre (-27.3238, -5.6498) ccw
  arc A223 (-29.3026, -11.5266) -> (-28.5237, -5.635) centre (-54.8238, -5.1553) ccw
  arc A224 (-30.0995, -14.2886) -> (-26.8376, -17.2859) centre (-27.8432, -15.1068) ccw
  line L263 (-20.4798, -14.3517) -> (-26.8376, -17.2859)
  arc A225 (-19.8144, -13.5364) -> (-18.8637, -4.9324) centre (-54.8378, -5.3119) ccw
  arc A226 (-20.4798, -14.3517) -> (-19.8144, -13.5364) centre (-20.9826, -13.2622) ccw
  arc A227 (-18.8637, -4.9324) -> (-20.1796, -3.7505) centre (-20.0636, -4.9449) ccw
  arc A228 (-5.1574, -2.7317) -> (-6.254, -1.7468) centre (-6.1573, -2.7421) ccw
  line L264 (-12.3041, -2.3342) -> (-6.254, -1.7468)
  arc A229 (-12.3041, -2.3342) -> (-13.2074, -3.3172) centre (-12.2075, -3.3295) ccw
  arc A230 (-14.5205, -10.5285) -> (-13.2074, -3.3172) centre (-35.1203, -3.0522) ccw
  arc A231 (-14.5205, -10.5285) -> (-11.8023, -13.0263) centre (-12.6403, -11.2103) ccw
  line L265 (-6.5041, -10.5811) -> (-11.8023, -13.0263)
  arc A232 (-5.9496, -9.9017) -> (-5.1574, -2.7317) centre (-35.1557, -3.0458) ccw
  arc A233 (-6.5041, -10.5811) -> (-5.9496, -9.9017) centre (-6.9232, -9.6732) ccw
  line L266 (-1.7605, -1.3106) -> (2.2307, -0.9231)
  arc A234 (-1.7605, -1.3106) -> (-2.6637, -2.328) centre (-1.6639, -2.3059) ccw
  arc A235 (-2.9278, -7.2425) -> (-2.6637, -2.328) centre (-35.1423, -3.0465) ccw
  arc A236 (-2.9278, -7.2425) -> (-1.5172, -8.2796) centre (-1.9362, -7.3717) ccw
  arc A237 (2.6874, -6.3392) -> (3.2663, -5.4948) centre (2.2683, -5.4312) ccw
  arc A238 (3.2663, -5.4948) -> (3.3269, -1.8883) centre (-35.1492, -3.0459) ccw
  arc A239 (3.3269, -1.8883) -> (2.2307, -0.9231) centre (2.3273, -1.9184) ccw
  arc A240 (6.3039, -4.877) -> (6.3144, -1.4722) centre (-35.1557, -3.0458) ccw
  arc A241 (7.2171, -0.4389) -> (6.3144, -1.4722) centre (7.3137, -1.4343) ccw
  line L267 (7.2171, -0.4389) -> (16.6808, 0.4799)
  arc A242 (6.3039, -4.877) -> (7.2118, -5.917) centre (7.3029, -4.9211) ccw
  line L268 (16.6687, -6.782) -> (7.2118, -5.917)
  arc A243 (16.6687, -6.782) -> (17.7585, -5.8353) centre (16.7598, -5.7861) ccw
  arc A244 (17.7585, -5.8353) -> (17.7766, -0.473) centre (-40.6706, -2.9578) ccw
  arc A245 (17.7766, -0.473) -> (16.6808, 0.4799) centre (16.7775, -0.5154) ccw
  line L269 (2.6874, -6.3392) -> (-1.5172, -8.2796)
  line L270 (-29.3026, -11.5266) -> (-30.0995, -14.2886)
  line L271 (-50.9967, 34.8873) -> (-50.9967, 36.3873)
  line L272 (-38.9967, 36.8873) -> (-38.9967, 37.8873)
  line L273 (-113.2523, 37.9487) -> (-114.7523, 37.9487)
  line L274 (-108.2523, 37.9487) -> (-106.7523, 37.9487)
  line L275 (-106.2523, 42.9487) -> (-105.2523, 42.9487)
  line L276 (-41.0445, 18.2036) -> (-58.6262, 16.9126)
  line L277 (-41.0445, 18.2036) -> (-58.6262, 16.9126)
  line L278 (-41.0445, 18.2036) -> (-58.6262, 16.9126)
  line L279 (-41.0445, 18.2036) -> (-58.6262, 16.9126)
  line L280 (-41.0445, 18.2036) -> (-62.9927, 16.5919)
  line L281 (-41.0445, 18.2036) -> (-58.6262, 16.9126)
  line L282 (-41.0445, 18.2036) -> (-58.6262, 16.9126)
  line L283 (-41.0445, 18.2036) -> (-58.6262, 16.9126)
  line L284 (-41.0445, 18.2036) -> (-58.6262, 16.9126)
  line L285 (-41.0445, 18.2036) -> (-58.6262, 16.9126)
  arc A246 (-40.1229, 19.0989) -> (-39.7117, 25.5947) centre (-123.1871, 27.6189) ccw
  arc A247 (-41.0445, 18.2036) -> (-40.1229, 19.0989) centre (-41.1177, 19.2009) ccw
  arc A248 (-39.7117, 25.5947) -> (-40.7114, 26.6189) centre (-40.7114, 25.6189) ccw
  line L286 (-40.7114, 26.6189) -> (-60.6957, 26.6189)
  arc A249 (-64.0519, 17.7563) -> (-62.9927, 16.5919) centre (-63.066, 17.5892) ccw
  line L287 (-60.6957, 26.6189) -> (-62.2338, 26.6189)
  arc A250 (-64.0519, 17.7563) -> (-63.233, 25.6575) centre (-124.6871, 28.0336) ccw
  arc A251 (-62.2338, 26.6189) -> (-63.233, 25.6575) centre (-62.2338, 25.6189) ccw
  arc A252 (-86.6984, 35.0217) -> (-85.7122, 38.078) centre (-117.0972, 46.5178) ccw
  arc A253 (-89.8905, 33.877) -> (-88.2189, 38.3912) centre (-117.0972, 46.5178) ccw
  arc A254 (-80.4624, 34.6799) -> (-79.8395, 36.8169) centre (-117.0972, 46.5178) ccw
  line L288 (-90.7241, 33.301) -> (-92.0131, 33.2064)
  line L289 (-90.7241, 33.301) -> (-92.0131, 33.2064)
  line L290 (-90.7241, 33.301) -> (-92.0131, 33.2064)
  line L291 (-90.7241, 33.301) -> (-92.0131, 33.2064)
  line L292 (-90.7241, 33.301) -> (-92.0131, 33.2064)
  line L293 (-90.7241, 33.301) -> (-92.0131, 33.2064)
  line L294 (-90.7241, 33.301) -> (-92.0131, 33.2064)
  line L295 (-90.7241, 33.301) -> (-92.0131, 33.2064)
  line L296 (-90.7241, 33.301) -> (-92.0131, 33.2064)
  line L297 (-81.3407, 33.9901) -> (-85.6898, 33.6707)
  line L298 (-81.3407, 33.9901) -> (-85.6898, 33.6707)
  line L299 (-81.3407, 33.9901) -> (-85.6898, 33.6707)
  line L300 (-81.3407, 33.9901) -> (-85.6898, 33.6707)
  line L301 (-81.3407, 33.9901) -> (-85.6898, 33.6707)
  line L302 (-81.3407, 33.9901) -> (-85.6898, 33.6707)
  line L303 (-81.3407, 33.9901) -> (-85.6898, 33.6707)
  line L304 (-81.3407, 33.9901) -> (-85.6898, 33.6707)
  line L305 (-81.3407, 33.9901) -> (-85.6898, 33.6707)
  line L306 (-84.5596, 38.8007) -> (-80.6203, 38.0513)
  arc A255 (-81.3407, 33.9901) -> (-80.4624, 34.6799) centre (-81.4139, 34.9874) ccw
  line L307 (-81.3407, 33.9901) -> (-85.6898, 33.6707)
  line L308 (-92.2961, 33.2259) -> (-96.0105, 34.0227)
  arc A256 (-97.3869, 36.8584) -> (-96.1092, 40.091) centre (-117.0972, 46.5178) ccw
  arc A257 (-97.3869, 36.8584) -> (-96.0105, 34.0227) centre (-95.591, 35.9782) ccw
  arc A258 (-92.2961, 33.2259) -> (-92.0131, 33.2064) centre (-92.0864, 34.2037) ccw
  line L309 (-90.7241, 33.301) -> (-92.0131, 33.2064)
  arc A259 (-79.8395, 36.8169) -> (-80.6203, 38.0513) centre (-80.8072, 37.0689) ccw
  line L310 (-94.9661, 40.7806) -> (-88.9946, 39.6445)
  arc A260 (-94.9661, 40.7806) -> (-96.1092, 40.091) centre (-95.153, 39.7982) ccw
  arc A261 (-88.2189, 38.3912) -> (-88.9946, 39.6445) centre (-89.1815, 38.6621) ccw
  arc A262 (-84.5596, 38.8007) -> (-85.7122, 38.078) centre (-84.7465, 37.8184) ccw
  arc A263 (-86.6984, 35.0217) -> (-85.6898, 33.6707) centre (-85.7631, 34.668) ccw
  arc A264 (-90.7241, 33.301) -> (-89.8905, 33.877) centre (-90.7974, 34.2983) ccw
  arc A265 (-74.6257, 37.3882) -> (-76.3606, 36.2812) centre (-74.906, 35.9146) ccw
  arc A266 (-76.6531, 35.1638) -> (-75.0921, 33.288) centre (-75.2019, 34.784) ccw
  arc A267 (-64.8982, 34.0366) -> (-64.813, 35.5213) centre (-64.9531, 34.7846) ccw
  arc A268 (63.3497, 5.1859) -> (64.4396, 6.1325) centre (63.4408, 6.1817) ccw
  line L311 (63.3497, 5.1859) -> (53.8928, 6.0509)
  arc A269 (64.4396, 6.1325) -> (64.4576, 11.4949) centre (6.0104, 9.0101) ccw
  arc A270 (64.4576, 11.4949) -> (63.3619, 12.4478) centre (63.4585, 11.4524) ccw
  line L312 (53.8981, 11.5289) -> (63.3619, 12.4478)
  arc A271 (52.9849, 7.0909) -> (52.9955, 10.4957) centre (11.5253, 8.9221) ccw
  arc A272 (53.8981, 11.5289) -> (52.9955, 10.4957) centre (53.9947, 10.5336) ccw
  arc A273 (52.9849, 7.0909) -> (53.8928, 6.0509) centre (53.9839, 7.0468) ccw
  line L313 (-81.2534, 67.7522) -> (-81.2534, 67.2522)
  line L314 (-81.2534, 69.7522) -> (-81.2534, 70.2522)
  line L315 (-120.7904, 67.7522) -> (-120.7904, 67.2522)
  line L316 (-120.7904, 69.7522) -> (-120.7904, 70.2522)
  line L317 (39.7, -51.2535) -> (39.7, -51.7535)
  line L318 (27.488, -49.2535) -> (39.7, -49.2535)
  line L319 (39.7, -49.2535) -> (39.7, -48.7535)
  line L320 (27.488, -45.2535) -> (39.7, -45.2535)
  line L321 (39.7, -45.2535) -> (39.7, -45.7535)
  line L322 (39.7, -43.2535) -> (39.7, -42.7535)
  line L323 (-74.1828, -67.805) -> (-73.7828, -67.805)
  line L324 (-76.1828, -62.305) -> (-76.1828, -67.805)
  line L325 (-76.1828, -67.805) -> (-76.5828, -67.805)
  line L326 (-35.7939, -43.5976) -> (-35.7939, -38.0976)
  line L327 (-35.7939, -38.0976) -> (-35.3939, -38.0976)
  line L328 (-37.7939, -38.0976) -> (-38.1939, -38.0976)
  line L329 (114.4127, 58.8312) -> (114.9235, 58.8312)
  line L330 (116.9397, 58.8287) -> (117.4289, 58.8275)
  line L331 (85.2029, -12.0118) -> (84.7029, -12.0118)
  line L332 (87.2029, -12.0118) -> (87.7029, -12.0118)
  line L333 (24.9941, 28.3361) -> (24.4941, 28.3361)
  line L334 (26.9941, 28.3361) -> (27.4941, 28.3361)
  line L335 (33.789, 16.9487) -> (92.4791, 33.2966)
  line L336 (116.9799, 9.8778) -> (-32.4689, -28.5336)
  line L337 (-76.6531, 35.1638) -> (-76.3606, 36.2812)
  line L338 (-75.0921, 33.288) -> (-64.8982, 34.0366)
  line L339 (-74.6257, 37.3882) -> (-64.813, 35.5213)
  line L340 (27.4941, 28.3361) -> (32.4941, 28.3361)
  arc A274 (32.4941, 28.3361) -> (36.0296, 31.8717) centre (32.0539, 32.3118) ccw
  line L341 (36.0296, 31.8717) -> (36.0296, 34.8717)
  arc A275 (37.0051, 39.7756) -> (36.0296, 34.8717) centre (46.0138, 35.4347) ccw
  line L342 (37.0051, 39.7756) -> (40.4492, 48.0905)
  arc A276 (40.4492, 48.0905) -> (36.5313, 49.3848) centre (39.5652, 51.9916) ccw
  line L343 (-114.7523, 37.9487) -> (-114.7523, 42.9487)
  line L344 (-114.7523, 42.9487) -> (-115.2523, 42.9487)
  line L345 (-106.7523, 37.9487) -> (-106.7523, 42.9487)
  line L346 (-106.7523, 42.9487) -> (-106.2523, 42.9487)
  line L347 (-50.9967, 36.3873) -> (-38.9967, 36.3873)
  line L348 (-38.9967, 36.3873) -> (-38.9967, 36.8873)
  line L349 (95.4791, 35.8778) -> (95.4791, 37.3778)
  line L350 (99.4807, 35.8778) -> (99.4807, 37.3778)
  line L351 (95.4791, 37.3778) -> (95.4791, 37.4038)
  line L352 (99.4807, 37.3778) -> (99.4807, 37.4038)
  line L353 (27.488, -45.2535) -> (27.488, -43.7535)
  line L354 (27.488, -43.7535) -> (39.7, -43.7535)
  line L355 (39.7, -43.7535) -> (39.7, -43.2535)
  line L356 (27.488, -49.2535) -> (27.488, -50.7535)
  line L357 (27.488, -50.7535) -> (39.7, -50.7535)
  line L358 (39.7, -50.7535) -> (39.7, -51.2535)
  line L359 (-35.7939, -43.5976) -> (-37.2939, -43.5976)
  line L360 (-37.2939, -43.5976) -> (-37.2939, -38.0976)
  line L361 (-37.2939, -38.0976) -> (-37.7939, -38.0976)
  line L362 (-76.1828, -62.305) -> (-74.6828, -62.305)
  line L363 (-74.6828, -62.305) -> (-74.6828, -67.805)
  line L364 (-74.6828, -67.805) -> (-74.1828, -67.805)
  line L365 (85.4529, -17.0118) -> (85.4529, -12.0118)
  line L366 (85.4529, -12.0118) -> (85.2029, -12.0118)
  line L367 (86.9529, -17.0118) -> (86.9529, -12.0118)
  line L368 (86.9529, -12.0118) -> (87.2029, -12.0118)
  line L369 (86.9529, -17.0118) -> (85.4529, -17.0118)
  circle A277 centre (76.9602, -40.3246) radius 1.525
  arc A278 (78.4852, -35.3246) -> (78.4852, -45.3246) centre (78.4852, -40.3246) ccw
  line L370 (82.4852, -35.3246) -> (78.4852, -35.3246)
  line L371 (86.2477, -35.3246) -> (87.0101, -35.3246)
  line L372 (87.0101, -35.3246) -> (91.0101, -35.3246) construction
  line L373 (78.4852, -45.3246) -> (91.0101, -45.3246)
  arc A279 (91.0101, -45.3246) -> (91.0101, -35.3246) centre (91.0101, -40.3246) ccw
  line L374 (87.0101, -35.3246) -> (91.0101, -35.3246)
  line L375 (83.7477, -35.3246) -> (83.2477, -35.3246)
  line L376 (85.7477, -35.3246) -> (86.2477, -35.3246)
  line L377 (82.4852, -35.3246) -> (83.2477, -35.3246)
  line L378 (85.4977, -40.3246) -> (83.9977, -40.3246)
  line L379 (83.9977, -40.3246) -> (83.9977, -35.3246)
  line L380 (85.4977, -40.3246) -> (85.4977, -35.3246)
  line L381 (85.4977, -35.3246) -> (85.7477, -35.3246)
  line L382 (83.9977, -35.3246) -> (83.7477, -35.3246)
  circle A280 centre (92.5351, -40.3246) radius 1.525
  line L383 (115.1735, 52.3219) -> (115.1735, 58.8312)
  line L384 (115.1735, 58.8312) -> (114.9235, 58.8312)
  line L385 (116.6735, 52.3219) -> (116.6735, 58.8287)
  line L386 (116.6735, 58.8287) -> (116.9397, 58.8287)
  line L387 (115.1735, 52.3219) -> (116.6735, 52.3219)
  line L388 (76.5441, 68.5821) -> (91.2573, 68.5821)
  line L389 (76.5441, 70.0821) -> (91.2573, 70.0821)
  line L390 (76.5441, 70.0821) -> (76.5441, 68.5821)
  arc A281 (91.2573, 70.0821) -> (92.0419, 71.8659) centre (90.0508, 71.6772) ccw
  arc A282 (92.0263, 66.8987) -> (91.2573, 68.5821) centre (90.029, 67.0037) ccw
  line L391 (-64.9559, 68.5821) -> (-57.4559, 68.5821)
  line L392 (-64.9559, 70.0821) -> (-57.4559, 70.0821)
  line L393 (-57.4559, 70.0821) -> (-57.4559, 68.5821)
  line L394 (-64.9559, 70.0821) -> (-64.9559, 68.5821)
  line L395 (26.7441, 34.8361) -> (26.7441, 28.3361)
  line L396 (26.7441, 28.3361) -> (26.9941, 28.3361)
  line L397 (25.2441, 34.8361) -> (25.2441, 28.3361)
  line L398 (25.2441, 28.3361) -> (24.9941, 28.3361)
  line L399 (25.2441, 34.8361) -> (26.7441, 34.8361)
  line L400 (-87.2534, 68.0022) -> (-81.2534, 68.0022)
  line L401 (-81.2534, 68.0022) -> (-81.2534, 67.7522)
  line L402 (-114.7904, 68.0022) -> (-120.7904, 68.0022)
  line L403 (-120.7904, 68.0022) -> (-120.7904, 67.7522)
  line L404 (-114.7904, 69.5022) -> (-120.7904, 69.5022)
  line L405 (-120.7904, 69.5022) -> (-120.7904, 69.7522)
  line L406 (-114.7904, 69.5022) -> (-114.7904, 68.0022)
  line L407 (-87.2534, 69.5022) -> (-81.2534, 69.5022)
  line L408 (-81.2534, 69.5022) -> (-81.2534, 69.7522)
  line L409 (-87.2534, 69.5022) -> (-87.2534, 68.0022)
  point P0 (0, 0)
  point P1 (48.3159, -27.9846)
  point P2 (15.9585, 31.8717)
  point P3 (-12.85, -51.3363)
  point P4 (-9.7016, -56.0072)
  point P5 (-6.9772, -57.0785)
  point P6 (18.6723, -56.1321)
  point P7 (31.0417, -56.1321)
  point P8 (33.7, -58.0785)
  point P9 (33.7, -36.4285)
  point P10 (28.9204, -39.2535)
  point P11 (16.4833, -37.4285)
  point P12 (-11.5744, -40.2419)
  point P13 (21.55, -51.2535)
  point P14 (20.55, -50.2535)
  point P15 (23.488, -43.2535)
  point P16 (24.488, -50.2535)
  point P17 (-40.8797, -38.6834)
  point P18 (-69.0752, -38.7415)
  point P19 (-80.6609, -43.6557)
  point P20 (-75.1609, -49.1557)
  point P21 (-69.0752, -48.57)
  point P22 (-31.7939, -40.0976)
  point P23 (-57.5769, -44.6799)
  point P24 (-52.5769, -44.6799)
  point P25 (-53.5769, -45.6799)
  point P26 (-46.268, -45.5976)
  point P27 (-47.268, -44.5976)
  point P28 (-66.9654, -45.7185)
  point P29 (-67.9654, -44.7185)
  point P30 (-67.9654, -42.7185)
  point P31 (-66.9654, -41.7185)
  point P32 (-63.9654, -41.7185)
  point P33 (-42.6541, -57.3458)
  point P34 (-71.097, -67.2192)
  point P35 (-50.7166, -60.152)
  point P36 (-46.7166, -61.152)
  point P37 (-46.7166, -63.152)
  point P38 (-50.7166, -64.152)
  point P39 (-51.7166, -63.152)
  point P40 (-60.1358, -60.2237)
  point P41 (-56.1358, -63.2237)
  point P42 (-57.1358, -64.2237)
  point P43 (-60.1358, -64.2237)
  point P44 (-65.7689, -60.305)
  point P45 (-65.7689, -64.305)
  point P46 (92.9791, 35.8778)
  point P47 (121.9799, 14.8778)
  point P48 (102.4799, 28.1985)
  point P49 (105.0023, 32.792)
  point P50 (100.9807, 39.1038)
  point P51 (93.9807, 37.7038)
  point P52 (95.4791, 37.4038)
  point P53 (-64.0519, 17.7563)
  point P54 (-63.233, 25.6575)
  point P55 (-40.7114, 26.6189)
  point P56 (-39.7117, 25.5947)
  point P57 (-40.1229, 19.0989)
  point P58 (-28.0267, 10.8747)
  point P59 (-18.5584, 8.835)
  point P60 (-20.5643, 3.4179)
  point P61 (-13.6957, 2.4536)
  point P62 (-15.0721, 5.2892)
  point P63 (-13.7944, 8.5218)
  point P64 (-6.6798, 8.0753)
  point P65 (-5.9041, 6.8221)
  point P66 (-7.5757, 2.3078)
  point P67 (20.3528, 5.0861)
  point P68 (21.1717, 12.9873)
  point P69 (43.6933, 13.9487)
  point P70 (44.693, 12.9245)
  point P71 (44.2818, 6.4287)
  point P72 (-92.2961, 33.2259)
  point P73 (-96.1092, 40.091)
  point P74 (-88.9946, 39.6445)
  point P75 (-88.2189, 38.3912)
  point P76 (-89.8905, 33.877)
  point P77 (-4.3836, 3.4526)
  point P78 (-3.3974, 6.5089)
  point P79 (2.4754, 5.2478)
  point P80 (1.8524, 3.1107)
  point P81 (106.3814, 13.1703)
  point P82 (106.3814, 16.5854)
  point P83 (107.4546, 17.5827)
  point P84 (112.0363, 14.1292)
  point P85 (-28.7231, 25.6842)
  point P86 (-19.1376, 24.8708)
  point P87 (-18.5493, 23.9983)
  point P88 (-18.3863, 15.3434)
  point P89 (-12.3041, -2.3342)
  point P90 (-6.254, -1.7468)
  point P91 (-5.9496, -9.9017)
  point P92 (17.7585, -5.8353)
  point P93 (6.3039, -4.877)
  point P94 (6.3144, -1.4722)
  point P95 (17.7766, -0.473)
  point P96 (-27.4398, -4.4554)
  point P97 (53.8981, 11.5289)
  point P98 (64.4576, 11.4949)
  point P99 (64.4396, 6.1325)
  point P100 (53.8928, 6.0509)
  point P101 (52.9849, 7.0909)
  point P102 (52.9955, 10.4957)
  point P103 (6.372, 9.6041)
  point P104 (6.6716, 12.9958)
  point P105 (18.166, 12.9067)
  point P106 (17.6954, 7.565)
  point P107 (-12.9006, 13.2197)
  point P108 (-13.5514, 20.5207)
  point P109 (-5.5636, 19.8429)
  point P110 (-5.0732, 19.1157)
  point P111 (-4.9374, 11.9034)
  point P112 (-2.4908, 11.2742)
  point P113 (-2.3062, 16.1924)
  point P114 (3.7029, 13.8877)
  point P115 (3.4347, 10.2907)
  point P116 (-85.7122, 38.078)
  point P117 (-80.6203, 38.0513)
  point P118 (-79.8395, 36.8169)
  point P119 (13.1579, 4.3013)
  point P120 (5.2668, 4.0718)
  point P121 (5.4595, 4.8078)
  point P122 (-69.9559, 70.3321)
  dimension "d65" = 3.1
  dimension "d66" = 3.1
  dimension "d67" = 5.5
  dimension "d68" = 3
  dimension "d69" = 3
  dimension "d70" = 5.5
  dimension "d71" = 3
  dimension "d72" = 3
  dimension "d73" = 2
  dimension "d74" = 3
  dimension "d75" = 2
  dimension "d76" = 3
  dimension "d77" = 2
  dimension "d78" = 3
  dimension "d79" = 2
  dimension "d80" = 3
  dimension "d81" = 140
  dimension "d82" = 140
  dimension "d83" = 3.1
  dimension "d84" = 3.1
  dimension "d85" = 8
  dimension "d86" = 8
  dimension "d87" = 3.1
  dimension "d88" = 3
  dimension "d89" = 2
  dimension "d90" = 2
  dimension "d91" = 2
  dimension "d92" = 2
  dimension "d93" = 3
  dimension "d94" = 2
  dimension "d95" = 2
  dimension "d96" = 2
  dimension "d97" = 2
  dimension "d98" = 3.1
  dimension "d99" = 3.1
  dimension "d100" = 5
  dimension "d101" = 5
  dimension "d102" = 4
  dimension "d103" = 3
  dimension "d104" = 5
  dimension "d105" = 10
  dimension "d106" = 9
  dimension "d107" = 4
  dimension "d108" = 3.1
  dimension "d109" = 3.1
  dimension "d110" = 6
  dimension "d111" = 6
  dimension "d112" = 2.5
  dimension "d113" = 6
  dimension "d114" = 6
  dimension "d115" = 2.5
  dimension "d116" = 1
  dimension "d117" = 1
  dimension "d118" = 22.2
  dimension "d119" = 22.2
  dimension "d120" = 3.1
  dimension "d121" = 3.1
  dimension "d122" = 3.1
  dimension "d123" = 3.1
  dimension "d124" = 3.1
  dimension "d125" = 3.1
  dimension "d126" = 3.1